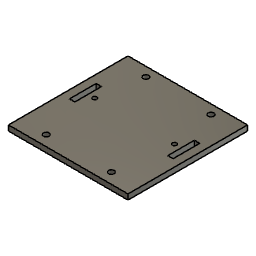
monitor_connect_plate (Autodesk Fusion 360 design; units mm, degrees)
Autodesk Fusion 360 part; units mm, degrees
note: some values were not read from the file. Set by a fixed rule: the direction of a hole.
sketch "スケッチ1" plane through (0, 0, 0) normal (0, 1, 0) x (1, 0, 0)
  line L0 (-45, 0) -> (45, 0)
  line L1 (45, 0) -> (45, 90)
  line L2 (45, 90) -> (-45, 90)
  line L3 (-45, 90) -> (-45, 0)
  line L4 (-39, 60) -> (-35, 60)
  line L5 (-35, 60) -> (-35, 40)
  line L6 (-35, 40) -> (-39, 40)
  line L7 (-39, 40) -> (-39, 60)
  line L8 (35, 60) -> (39, 60)
  line L9 (39, 60) -> (39, 40)
  line L10 (39, 40) -> (35, 40)
  line L11 (35, 40) -> (35, 60)
  line L12 (-24.5, 83) -> (24.5, 83)
  line L13 (24.5, 83) -> (24.5, 8)
  line L14 (24.5, 8) -> (-24.5, 8)
  line L15 (-24.5, 8) -> (-24.5, 83)
  line L16 (-35, 50) -> (-30, 50)
  line L17 (35, 50) -> (30, 50)
  point P0 (0, 8)
  dimension "d1" = 90
  dimension "d2" = 90
  dimension "d3" = 40
  dimension "d4" = 20
  dimension "d5" = 4
  dimension "d6" = 35
  dimension "d7" = 35
  dimension "d8" = 49
  dimension "d9" = 75
  dimension "d10" = 8
  dimension "d16" = 5
  dimension "d17" = 5
  constraint horizontal L0
  constraint vertical L1
  constraint horizontal L2
  constraint vertical L3
  constraint midpoint origin L0
  constraint horizontal L4
  constraint vertical L5
  constraint horizontal L6
  constraint vertical L7
  constraint horizontal L8
  constraint vertical L9
  constraint horizontal L10
  constraint vertical L11
  constraint equal L4 L8
  constraint collinear L4 L8
  constraint collinear L6 L10
  constraint horizontal L12
  constraint vertical L13
  constraint horizontal L14
  constraint vertical L15
  constraint midpoint L14 P0
  constraint vertical origin P0
  constraint midpoint L5 L16.start
  constraint perpendicular L5 L16
  constraint midpoint L11 L17.start
  constraint perpendicular L11 L17
  measures "d1" distance of L0.start L0.end
  measures "d2" distance of L0.end L1.end
  measures "d3" distance of L0 L10
  measures "d4" distance of L8.end L9.end
  measures "d5" distance of L8.start L8.end
  measures "d6" distance of origin L11
  measures "d7" distance of origin L5
  measures "d8" distance of L12.start L12.end
  measures "d9" distance of L12.end L13.end
  measures "d10" distance of L0 L14
  measures "d16" distance of L16.start L16.end
  measures "d17" distance of L17.start L17.end
extrude "押し出し1" add sketch "スケッチ1" along normal blind 4 contours L0 L1 L2 L3 | L12 L13 L14 L15
hole "穴1" at (-24.5, 0, -8) at (24.5, 0, -8) at (24.5, 0, -83) at (-24.5, 0, -83) direction (0, 1, 0) diameter 4.3 depth 4 tip angle 118
hole "穴2" at (-30, 0, -50) at (30, 0, -50) direction (0, 1, 0) diameter 3.2 end through all
